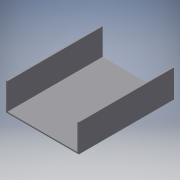
# Autodesk Inventor part: C Chanel
Saved by Autodesk Inventor 2017 (Build 210142000, 142)
## iProperties
Created: 2019-02-05
Part Number: C Chanel
Material: Generic
Document SubType Name: Modeling
Designer: S346795925
Density: 1 g/cm^3
Appearance: Default
Author: S346795925
Autodesk Inventor part; units mm, degrees
ref_plane "YZ Plane" through (0, 0, 0) normal (1, 0, 0) x (0, 1, 0)
ref_plane "XZ Plane" through (0, 0, 0) normal (0, 1, 0) x (-1, 0, 0)
ref_plane "XY Plane" through (0, 0, 0) normal (0, 0, 1) x (1, 0, 0)
sketch "Sketch1" plane through (0, 0, 0) normal (0, 0, 1) x (1, 0, 0)
  line L0 (0, 0) -> (0, -63.5)
  line L1 (0, -63.5) -> (168.275, -63.5)
  line L2 (168.275, -63.5) -> (168.275, 0)
  line L3 (-3.175, 0) -> (-3.175, -66.675)
  line L4 (-3.175, -66.675) -> (171.45, -66.675)
  line L5 (171.45, -66.675) -> (171.45, 0)
  line L6 (0, 0) -> (-3.175, 0)
  line L7 (168.275, 0) -> (171.45, 0)
  dimension "d0" = 63.5
  dimension "d2" = 168.275
  dimension "d3" = 90
  dimension "d4" = 3.175
  constraints: 16 end point, 5 perpendicular, 2 collinear, 1 vertical, 2 other
  measures "d0" distance of L0.start L0.end
  measures "d2" distance of L0.end L1.end
  measures "d3" angle of L1 L0
  measures "d4" distance between parallel lines of L0 L3
extrude "Extrusion1" add sketch "Sketch1" along normal blind 228.6
body "Solid1"
